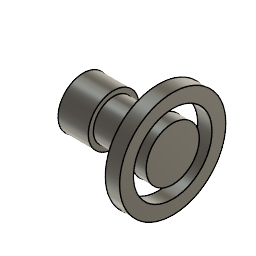
Day 7 (Autodesk Fusion 360 design; units mm, degrees)
Autodesk Fusion 360 part; units mm, degrees
sketch "Sketch1" plane through (0, 0, 0) normal (0, 1, 0) x (1, 0, 0)
  line L0 (-125, 0) -> (145, 0) construction
  line L1 (-114.9, 0) -> (-114.9, -19)
  line L2 (-114.9, 0) -> (-114.9, -25)
  line L3 (-114.9, -19) -> (-90.9, -19)
  line L4 (-114.9, -25) -> (-84.9, -25)
  line L5 (-90.9, -19) -> (-90.9, -15)
  line L6 (-84.9, -25) -> (-84.9, -20)
  line L7 (-84.9, -20) -> (-40.7, -20)
  line L8 (-40.7, -20) -> (-40.7, 0) construction
  line L9 (-40.7, -20) -> (-40.7, -52.5)
  line L10 (-40.7, -52.5) -> (-26.5, -52.5)
  line L11 (-26.5, -52.5) -> (-26.5, 0)
  line L12 (-26.5, 0) -> (-30, 0)
  line L13 (-30, 0) -> (-30, -15)
  line L14 (-26.5, -18) -> (-27, -18)
  line L15 (-27, -18) -> (-30, -15)
  line L16 (-90.9, -15) -> (-26.5, -15)
  line L17 (-40.7, 0) -> (-40.7, -32.5) construction
  line L18 (-40.7, -32.5) -> (-12.9644, -32.5) construction
  line L19 (-40.7, -38.75) -> (-26.5, -38.75)
  line L20 (-40.7, -26.25) -> (-26.5, -26.25)
  point P0 (-30, -18)
  dimension "d5" = 19
  dimension "d6" = 25
  dimension "d7" = 24
  dimension "d8" = 30
  dimension "d9" = 4
  dimension "d10" = 5
  dimension "d11" = 44.2
  dimension "d12" = 32.5
  dimension "d13" = 14.2
  dimension "d14" = 3.5
  dimension "d15" = 3
  dimension "d16" = 3
  dimension "d17" = 32.5
  dimension "d18" = 6.25
  constraint horizontal L0
  constraint coincident L0 L1.start
  constraint perpendicular L0 L1
  constraint perpendicular L0 L2
  constraint perpendicular L2 L3
  constraint perpendicular L2 L4
  constraint perpendicular L3 L5
  constraint perpendicular L4 L6
  constraint perpendicular L6 L7
  constraint coincident L0 L8.end
  constraint perpendicular L0 L8
  constraint perpendicular L7 L9
  constraint perpendicular L9 L10
  constraint coincident L0 L11.end
  constraint perpendicular L0 L11
  constraint perpendicular L11 L12
  constraint perpendicular L0 L13
  constraint coincident L11 L14.start
  constraint perpendicular L13 L14
  constraint coincident L14 P0
  constraint coincident L13 P0
  constraint coincident L11 L16.end
  constraint perpendicular L11 L16
  constraint perpendicular L7 L17
  constraint perpendicular L11 L18
  constraint coincident L9 L19.start
  constraint coincident L11 L19.end
  constraint perpendicular L11 L19
  constraint symmetric L18 L19.start L20.start
  constraint symmetric L18 L19.end L20.end
  measures "d5" distance of L1.start L1.end
  measures "d6" distance of L1.start L2.end
  measures "d7" distance of L1.end L3.end
  measures "d8" distance of L2.end L4.end
  measures "d9" distance of L3.end L5.end
  measures "d10" distance of L4.end L6.end
  measures "d11" distance of L6.end L7.end
  measures "d12" distance of L7.end L9.end
  measures "d13" distance of L9.end L10.end
  measures "d14" distance of L11.end L12.end
  measures "d15" distance of L14.end P0
  measures "d16" distance of L13.end P0
  measures "d17" distance of L8.end L17.end
  measures "d18" distance of L18 L19
revolve "Revolve1" add sketch "Sketch1" angle 360 about axis through (-125, 0, 0) along (1, 0, 0) contours L2 L3 L4 L5 L6 L7 L9 L11 L14 L15 L16 L20 | L11 L14 L15 L16 | L11 L12 L13 L16 | L9 L10 L11 L19 makes body 1 at (-31.2333, 5.2273, 52.2391) makes body 2 at (-50.3, 1.4935, 14.9255)
equation "d8 = 24 mm + 6 mm"
equation "d9 = 19 mm - 15 mm"
equation "d10 = 25 mm - 20 mm"
equation "d12 = ( 65 / 2 ) * 1 mm"
equation "d16 = d15"
equation "d17 = ( 65 / 2 ) * 1 mm"
equation "d18 = ( 12.5 / 2 ) * 1 mm"
